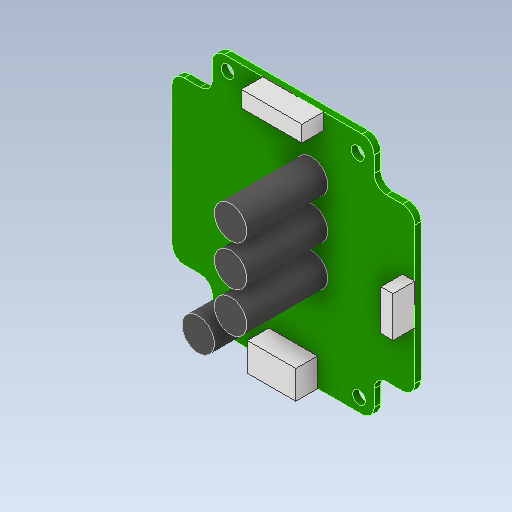
# Autodesk Inventor part: TMCM-1260_PCB
Saved by Autodesk Inventor 2021 (Build 250183000, 183)
## iProperties
Created: 2020-02-26
Part Number: TMCM-1260_PCB
Material: Generic
Document SubType Name: Modeling
Designer: Viktor Lindström
Density: 1 g/cm^3
Appearance: Default
Author: Viktor Lindström
Autodesk Inventor part; units mm, degrees
ref_plane "YZ Plane" through (0, 0, 0) normal (1, 0, 0) x (0, 1, 0)
ref_plane "XZ Plane" through (0, 0, 0) normal (0, 1, 0) x (-1, 0, 0)
ref_plane "XY Plane" through (0, 0, 0) normal (0, 0, 1) x (1, 0, 0)
sketch "Sketch1" plane through (0, 0, 0) normal (0, 0, 1) x (1, 0, 0)
  line L0 (-30, -30) -> (30, -30)
  line L1 (30, -30) -> (30, 30)
  line L2 (30, 30) -> (-30, 30)
  line L3 (-30, 30) -> (-30, -30)
  line L4 (-30, -30) -> (30, 30) construction
  line L5 (30, -30) -> (-30, 30) construction
  point P0 (0, 0)
  dimension "d0" = 60
  dimension "d1" = 60
  constraints: 12 end point, 2 midpoint, 2 parallel, 1 horizontal, 1 perpendicular
  measures "d0" distance of L1.end L2.end
  measures "d1" distance of L0.end L1.end
extrude "Extrusion1" add sketch "Sketch1" along normal blind 1.6
sketch "Sketch2" plane through (0, 0, 1.6) normal (0, 0, 1) x (1, 0, 0)
  line L0 (-30, -30) -> (30, -30) construction
  line L1 (30, -30) -> (30, 30) construction
  line L2 (30, 30) -> (-30, 30) construction
  line L3 (-30, 30) -> (-30, -30) construction
  line L4 (-30, -30) -> (-20, -30)
  line L5 (-20, -30) -> (-20, -20)
  line L6 (-20, -20) -> (-30, -20)
  line L7 (-30, -20) -> (-30, -30)
  line L8 (-42, 0) -> (42, 0) construction
  line L9 (0, -42) -> (0, 42) construction
  line L10 (-30, 30) -> (-20, 30)
  line L11 (-20, 30) -> (-20, 20)
  line L12 (-20, 20) -> (-30, 20)
  line L13 (-30, 20) -> (-30, 30)
  line L14 (30, 30) -> (30, -30) construction
  line L15 (30, -30) -> (20, -30)
  line L16 (20, -30) -> (20, -20)
  line L17 (20, -20) -> (30, -20)
  line L18 (30, -20) -> (30, -30)
  line L19 (30, 30) -> (20, 30)
  line L20 (20, 30) -> (20, 20)
  line L21 (20, 20) -> (30, 20)
  line L22 (30, 20) -> (30, 30)
  point P0 (0, 0)
  dimension "d4" = 10
  dimension "d5" = 10
  constraints: 34 end point, 9 symmetric about line, 2 parallel, 1 horizontal, 1 perpendicular
  measures "d4" distance of L5.end L6.end
  measures "d5" distance of L4.end L5.end
extrude "Extrusion2" cut sketch "Sketch2" against normal blind 1.6
fillet "Fillet1" radius 3 12 edges at (30, 20, 0.8) (20, 20, 0.8) (20, 30, 0.8) (-20, 30, 0.8) (-20, 20, 0.8) (-30, 20, 0.8) (-30, -20, 0.8) (-20, -20, 0.8) (-20, -30, 0.8) (20, -30, 0.8) (20, -20, 0.8) (30, -20, 0.8)
sketch "Sketch3" plane through (0, 0, 1.6) normal (0, 0, 1) x (1, 0, 0)
  line L0 (-42, 0) -> (42, 0) construction
  line L1 (0, -42) -> (0, 42) construction
  circle A0 centre (16.25, -26.75) radius 1.6
  line L2 (-17, -30) -> (17, -30) construction
  line L3 (30, -17) -> (30, 17) construction
  circle A1 centre (-15.95, -25.4) radius 1.6
  circle A2 centre (-16.25, 26.75) radius 1.6
  circle A3 centre (15.95, 25.4) radius 1.6
  point P0 (0, 0)
  dimension "d9" = 3.25
  dimension "d10" = 13.75
  dimension "d11" = 3.2
  dimension "d12" = 3.2
  dimension "d13" = 3.2
  dimension "d14" = 3.2
  dimension "d15" = 4.6
  dimension "d16" = 45.95
  dimension "d17" = 56.75
  dimension "d18" = 46.25
  dimension "d19" = 55.4
  dimension "d20" = 14.05
  dimension "d41" = 52.15
  dimension "d42" = 0.3
  dimension "d43" = 32.2
  dimension "d44" = 32.2
  dimension "d45" = 52.15
  dimension "d46" = 1.35
  constraints: 4 centre point
  measures "d9" distance from line of L2 A0.centre
  measures "d10" distance from line of L3 A0.centre
  measures "d11" diameter of A0
  measures "d12" diameter of A1
  measures "d13" diameter of A2
  measures "d14" diameter of A3
  measures "d15" distance from line of L2 A1.centre
  measures "d16" distance from line of L3 A1.centre
  measures "d17" distance from line of L2 A2.centre
  measures "d18" distance from line of L3 A2.centre
  measures "d19" distance from line of L2 A3.centre
  measures "d20" distance from line of L3 A3.centre
  measures "d41" vertical distance of A2.centre A1.centre
  measures "d42" horizontal distance of A2.centre A1.centre
  measures "d43" horizontal distance of A1.centre A0.centre
  measures "d44" horizontal distance of A2.centre A3.centre
  measures "d45" vertical distance of A3.centre A0.centre
  measures "d46" vertical distance of A0.centre A1.centre
extrude "Extrusion3" cut sketch "Sketch3" against normal blind 1.6
sketch "Sketch4" plane through (0, 0, 1.6) normal (0, 0, 1) x (1, 0, 0)
  line L0 (-17, -30) -> (17, -30) projected
  line L1 (-6, -30) -> (6, -30)
  line L2 (6, -30) -> (6, -23)
  line L3 (6, -23) -> (-6, -23)
  line L4 (-6, -23) -> (-6, -30)
  line L5 (17, 30) -> (-17, 30) projected
  line L6 (-7.5, 30) -> (7.5, 30)
  line L7 (7.5, 30) -> (7.5, 26)
  line L8 (7.5, 26) -> (-7.5, 26)
  line L9 (-7.5, 26) -> (-7.5, 30)
  line L10 (30, -17) -> (30, 17) projected
  line L11 (30, -17) -> (30, 17) projected
  line L12 (30, -5) -> (27, -5)
  line L13 (27, -5) -> (27, 5)
  line L14 (27, 5) -> (30, 5)
  line L15 (30, 5) -> (30, -5)
  point P0 (0, 0)
  dimension "d23" = 12
  dimension "d24" = 7
  dimension "d25" = 6
  dimension "d26" = 15
  dimension "d27" = 7.5
  dimension "d28" = 4
  dimension "d29" = 3
  dimension "d30" = 5
  dimension "d31" = 10
  constraints: 24 end point, 6 parallel, 3 horizontal, 3 perpendicular, 3 point on line
  measures "d23" distance between parallel lines of L2 L4
  measures "d24" distance between parallel lines of L0 L3
  measures "d25" distance from line of point (0, 0) L4
  measures "d26" distance of L7.end L8.end
  measures "d27" distance from line of point (0, 0) L9
  measures "d28" distance between parallel lines of L5 L8
  measures "d29" distance between parallel lines of L15 L13
  measures "d30" distance from line of point (0, 0) L12
  measures "d31" distance between parallel lines of L14 L12
extrude "Extrusion4" add sketch "Sketch4" along normal blind 5.35 separate body
sketch "Sketch5" plane through (0, 0, 1.6) normal (0, 0, 1) x (1, 0, 0)
  circle A0 centre (-3.4878, -13.1301) radius 4
  circle A1 centre (4.5122, -5.1301) radius 4
  circle A2 centre (4.5122, 4.8699) radius 4
  circle A3 centre (4.5122, 14.8699) radius 4
  line L0 (4.5122, -5.1301) -> (4.5122, 14.6748) construction
  point P0 (0, 0)
  dimension "d34" = 10
  dimension "d35" = 10
  dimension "d36" = 8
  dimension "d37" = 8
  dimension "d38" = 8
  constraints: 4 centre point, 3 equal radius, 2 end point, 1 vertical
  measures "d34" distance of A2.centre L0.start
  measures "d35" distance of A3.centre A2.centre
  measures "d36" horizontal distance of A0.centre L0.start
  measures "d37" horizontal distance of L0.start A0.centre
  measures "d38" diameter of A1
extrude "Extrusion5" add sketch "Sketch5" along normal blind 20 separate body
equation "\"d5\" = d4"
equation "\"d12\" = d11"
equation "\"d13\" = d12"
equation "\"d14\" = d13"
equation "\"d30\" = 0.5 * d31"
body "Solid1"
body "Solid2"
body "Solid3"
